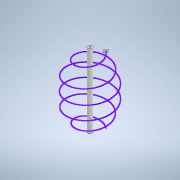
# Autodesk Inventor part: cir
Saved by Autodesk Inventor 2022 (Build 260153000, 153)
## iProperties
Created: 2023-03-25
Part Number: cir
Material: 一般
Document SubType Name: Modeling
Designer: JOU
Density: 1 g/cm^3
Appearance: 預設
Mass: 314.159 g
Surface Area: 640.885 cm^2
Volume: 314.159 cm^3
Author: JOU
Autodesk Inventor part; units mm, degrees
ref_plane "YZ Plane" through (0, 0, 0) normal (1, 0, 0) x (0, 1, 0)
ref_plane "XZ Plane" through (0, 0, 0) normal (0, 1, 0) x (-1, 0, 0)
ref_plane "XY Plane" through (0, 0, 0) normal (0, 0, 1) x (1, 0, 0)
sketch "草圖1" plane through (0, 0, 0) normal (0, 1, 0) x (-1, 0, 0)
  circle A0 centre (0, 0) radius 5
  circle A1 centre (0, 0) radius 15
  dimension "d0" = 10
  dimension "d1" = 30
  constraints: 2 centre point, 2 coincident
  measures "d0" diameter of A0
  measures "d1" diameter of A1
extrude "擠出1" add sketch "草圖1" along normal blind 500
sketch3d "3D 草圖1"
sketch3d "3D 草圖2"
sketch3d "3D 草圖3"
sketch3d "3D 草圖5"
sketch3d "3D 草圖6"
sketch3d "3D 草圖7"
ref_plane "工作平面2" through (43.768, 465.3652, -63.5362) normal (-0.8064, 0.1825, -0.5625) x (-0.2208, -0.9753, 0)
